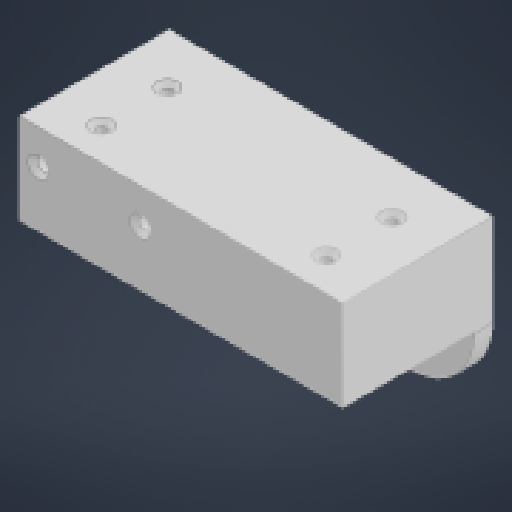
# Autodesk Inventor part: PRINTED right z mount 2
Saved by Autodesk Inventor 2024 (Build 280153000, 153)
## iProperties
Created: 2024-07-29
Part Number: PRINTED right z mount 2
Material: Generic
Document SubType Name: Modeling
Designer: mateu
Density: 1 g/cm^3
Appearance: Default
Author: mateu
Autodesk Inventor part; units mm, degrees
ref_plane "YZ Plane" through (0, 0, 0) normal (1, 0, 0) x (0, 1, 0)
ref_plane "XZ Plane" through (0, 0, 0) normal (0, 1, 0) x (-1, 0, 0)
ref_plane "XY Plane" through (0, 0, 0) normal (0, 0, 1) x (1, 0, 0)
sketch "Sketch1" plane through (0, 0, 0) normal (0, 0, 1) x (1, 0, 0)
  arc A0 (14.1427, -15.2387) -> (13.4175, -14.0632) centre (13.1646, -15.0307) ccw projected
  line L0 (13.4175, -14.0632) -> (9.4746, -13.0327) projected
  arc A1 (9.4746, -13.0327) -> (0.5427, -12.0878) centre (1.8884, -42.0576) ccw projected
  arc A2 (1.3475, 12.0247) -> (0.5427, -12.0878) centre (0, 0) ccw projected
  arc A3 (1.3475, 12.0247) -> (10.3225, 12.3719) centre (4.6883, 41.8381) ccw projected
  line L1 (10.3225, 12.3719) -> (21.175, 14.447) projected
  line L2 (21.175, 14.447) -> (21.175, 21.6191) projected
  line L3 (-21.175, 20.6809) -> (-21.175, -21.125) projected
  line L4 (-21.175, -21.125) -> (21.175, -21.125) projected
  line L5 (21.175, -21.125) -> (21.175, -16.0908) projected
  line L6 (21.175, -16.0908) -> (17.9879, -15.2578) projected
  arc A4 (17.9879, -15.2578) -> (16.7802, -15.9281) centre (17.735, -16.2253) ccw projected
  arc A5 (14.1427, -15.2387) -> (16.7802, -15.9281) centre (15.4774, -15.5226) ccw projected
  circle A6 centre (-15.4774, 15.5226) radius 1.3645 projected
  circle A7 centre (-15.5226, -15.4774) radius 1.3645 projected
  circle A8 centre (15.5226, 15.4774) radius 1.3645 projected
  circle A9 centre (57.9677, -1.9346) radius 4.2 projected
  circle A10 centre (57.9677, -1.9346) radius 19.1904
  line L7 (21.175, -21.125) -> (57.9677, -21.125)
  line L8 (21.175, 21.125) -> (77.1581, 21.125)
  line L9 (77.1581, 21.125) -> (77.1581, -1.9346)
  line L10 (-21.1741, 21.6809) -> (21.175, 21.6191) projected
  line L11 (-21.1741, 21.6809) -> (-21.1756, 20.6809) projected
  line L12 (-21.175, 20.6809) -> (-21.1756, 20.6809) projected
  point P0 (0, 0)
  point P1 (-21.175, 21.125)
  constraints: 6 end point, 2 point on circle, 2 tangent, 1 centre point, 1 coincident, 1 horizontal
extrude "Extrusion1" add sketch "Sketch1" along normal blind 5.5
sketch "Sketch2" plane through (0, 0, 5.5) normal (0, 0, 1) x (1, 0, 0)
  line L0 (77.1581, -1.9346) -> (77.1581, 21.125) projected
  line L1 (-21.175, 20.6809) -> (-21.175, -21.125) projected
  line L2 (-21.175, -21.125) -> (57.9677, -21.125) projected
  arc A0 (57.9677, -21.125) -> (77.1581, -1.9346) centre (57.9677, -1.9346) ccw projected
  circle A1 centre (15.5226, 15.4774) radius 1.3645 projected
  circle A2 centre (-15.5226, -15.4774) radius 1.3645 projected
  circle A3 centre (-15.4774, 15.5226) radius 1.3645 projected
  circle A4 centre (57.9677, -1.9346) radius 4.2 projected
  line L3 (110.8694, -1.8119) -> (-349.1301, -1.1403) projected
  line L4 (110.8699, -1.5119) -> (-349.1296, -0.8403)
  line L5 (21.175, 21.6191) -> (-21.1741, 21.6809) projected
  line L6 (-21.1741, 21.6809) -> (-21.1756, 20.6809) projected
  line L7 (-21.1756, 20.6809) -> (-21.175, 20.6809) projected
  line L8 (77.1581, 21.125) -> (21.175, 21.125) projected
  line L9 (21.175, 21.125) -> (21.175, 21.6191) projected
  point P0 (0, 0)
  point P1 (-21.175, -1.3191)
  point P2 (77.1581, -1.4626)
  dimension "d2" = 0.3
  constraints: 2 end point, 1 parallel
  measures "d2" distance between parallel lines of L3 L4
ref_plane "Work Plane1" through (-349.1377, -7.0016, 45.5) normal (0, 0, 1) x (0.9999989, -0.0014598, 0)
extrude "Extrusion2" add sketch "Sketch2" along normal up to surface (40 mm away) contours A0 L2 L1 L3 A4 L0 | L3 A4 L4 L0 | L4 A4 L1 L6 L5 L9 L8 L0 | L3 A4 L4 | A4 L3 | L4 A4 | L3 L1 L4 A4 | A2
sketch "Sketch3" plane through (-21.175, 26.125, 0) normal (0, 1, 0) x (1, 0, 0)
  line L0 (-327.9643, -38.4057) -> (-327.9643, -32.5943) projected
  line L1 (132.0352, -38.4057) -> (-327.9643, -38.4057) projected
  line L2 (132.0352, -38.4057) -> (132.0352, -32.5943) projected
  line L3 (132.0352, -32.5943) -> (-327.9643, -32.5943) projected
  line L4 (-327.9643, -18.4057) -> (-327.9643, -12.5943) projected
  line L5 (132.0352, -18.4057) -> (-327.9643, -18.4057) projected
  line L6 (132.0352, -18.4057) -> (132.0352, -12.5943) projected
  line L7 (132.0352, -12.5943) -> (-327.9643, -12.5943) projected
  line L8 (98.3331, 0) -> (98.3331, -45.5) projected
  line L9 (0, 0) -> (0, -45.5) projected
  point P0 (21.175, 0)
  point P1 (83.3331, -35.5)
  point P2 (83.3331, -35.5)
  point P3 (15, -15.5)
  point P4 (83.3331, -15.5)
  point P5 (15, -35.5)
  dimension "d8" = 15
  dimension "d9" = 15
  constraints: 2 coincident, 1 horizontal alignment, 1 vertical alignment
  measures "d8" distance from line of L8 point (83.333, -35.5)
  measures "d9" distance from line of L9 point (15, -15.5)
hole "Hole1" [suppressed]
sketch "Sketch4" plane through (-21.175, 26.125, 45.5) normal (0, 0, 1) x (1, 0, 0)
  circle A0 centre (36.6976, -10.6476) radius 1.3645 projected
  circle A1 centre (5.6976, -10.6024) radius 1.3645 projected
  circle A2 centre (5.6523, -41.6024) radius 1.3645 projected
  point P0 (21.175, -26.125)
hole "Hole2" at (15.5226, 15.4774, 45.5) at (-15.4774, 15.5226, 45.5) at (-15.5226, -15.4774, 45.5) direction (0, 0, -1) diameter 3.4 end through all countersink diameter 6.3 countersink angle 90 clearance for "Countersunk Flat Head Screw ISO 2009/7046" size "M3" standard "ISO"
sketch "Sketch5" plane through (0, 0, 0) normal (0, 0, -1) x (-1, 0, 0)
  arc A0 (-62.1677, -1.9346) -> (-62.1677, -1.9346) centre (-57.9677, -1.9346) ccw projected
  circle A1 centre (-57.9677, -1.9346) radius 8.1
  point P0 (0, 0)
  dimension "d24" = 16.2
  constraints: 1 centre point, 1 coincident
  measures "d24" diameter of A1
extrude "Extrusion3" cut sketch "Sketch5" against normal up to surface (5.5 mm away) contours A0 | A1
sketch "Sketch6" plane through (0, 0, 5.5) normal (0, 0, 1) x (1, 0, 0)
  circle A0 centre (15.4774, -15.5226) radius 2.3806 projected
  circle A1 centre (-15.5226, -15.4774) radius 1.7 projected
  point P0 (0, 0)
hole "Hole3" at (15.4774, -15.5226, 5.5) at (-15.5226, -15.4774, 5.5) direction (0, 0, -1) diameter 3.4 end through all countersink diameter 6.3 countersink angle 90 clearance for "Countersunk Flat Head Screw ISO 2009/7046" size "M3" standard "ISO"
sketch "Sketch7" plane through (77.1581, -1.9346, 5.5) normal (1, 0, 0) x (0, 0, -1)
  circle A0 centre (-20, 14.2658) radius 4.5 projected
  point P0 (5.5, 1.9346)
hole "Hole4" at (77.1581, 12.3312, 25.5) direction (-1, 0, 0) diameter 4.8 depth 20
body "Solid1"
